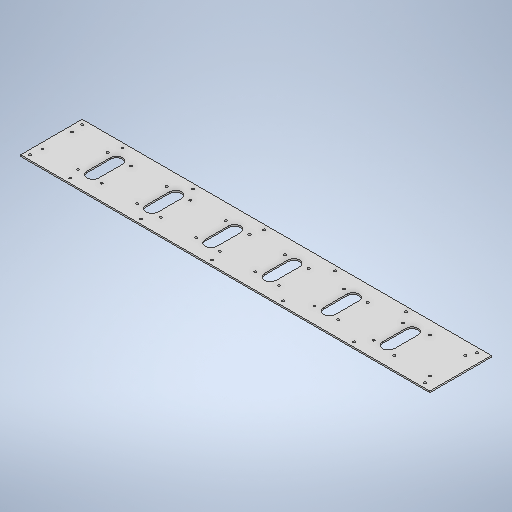
# Autodesk Inventor part: PCBMountingPlate
Saved by Autodesk Inventor 2025.1 (Build 291241000, 241)
## iProperties
Created: 2025-12-18
Part Number: PCBMountingPlate
Material: Generic
Document SubType Name: Modeling
Designer: Juxin
Density: 1 g/cm^3
Appearance: Default
Author: Juxin
Autodesk Inventor part; units mm, degrees
ref_plane "YZ Plane" through (0, 0, 0) normal (1, 0, 0) x (0, 1, 0)
ref_plane "XZ Plane" through (0, 0, 0) normal (0, 1, 0) x (-1, 0, 0)
ref_plane "XY Plane" through (0, 0, 0) normal (0, 0, 1) x (1, 0, 0)
sketch "Sketch1" plane through (0, 0, 0) normal (0, 1, 0) x (-1, 0, 0)
  line L0 (0, 0) -> (878.84, 0)
  line L1 (878.84, 0) -> (878.84, -66.04)
  line L2 (878.84, -66.04) -> (0, -66.04)
  line L3 (0, -66.04) -> (0, 0)
  line L4 (0, 0) -> (0, -20.32)
  line L5 (0, 0) -> (20.32, 0) construction
  line L6 (0, -20.32) -> (878.84, -20.32)
  line L7 (0, -10.16) -> (20.32, -10.16)
  line L8 (0, -10.16) -> (20.32, -10.16) construction
  circle A0 centre (20.32, -10.16) radius 2.54
  line L9 (20.32, -10.16) -> (172.72, -10.16)
  line L10 (20.32, -10.16) -> (172.72, -10.16) construction
  circle A1 centre (172.72, -10.16) radius 2.54
  line L11 (172.72, -10.16) -> (325.12, -10.16)
  circle A2 centre (325.12, -10.16) radius 2.54
  line L12 (325.12, -10.16) -> (477.52, -10.16)
  circle A3 centre (477.52, -10.16) radius 2.54
  line L13 (477.52, -10.16) -> (629.92, -10.16)
  circle A4 centre (629.92, -10.16) radius 2.54
  line L14 (629.92, -10.16) -> (782.32, -10.16)
  circle A5 centre (782.32, -10.16) radius 2.54
  line L15 (878.84, 0) -> (878.84, -10.16)
  line L16 (878.84, 0) -> (889, 0) construction
  line L17 (878.84, -10.16) -> (868.68, -10.16)
  circle A6 centre (868.68, -10.16) radius 2.54
  line L18 (0, 0) -> (0, -27.94)
  line L19 (0, 0) -> (27.94, 0) construction
  line L20 (0, -27.94) -> (27.94, -27.94)
  circle A7 centre (27.94, -27.94) radius 2.54
  line L21 (27.94, -27.94) -> (104.14, -27.94)
  line L22 (27.94, -27.94) -> (104.14, -27.94) construction
  circle A8 centre (104.14, -27.94) radius 2.54
  line L23 (104.14, -27.94) -> (129.54, -27.94)
  line L24 (142.24, -40.64) -> (142.24, -66.04)
  line L25 (142.24, -66.04) -> (116.84, -66.04)
  line L26 (116.84, -66.04) -> (116.84, -40.64)
  line L27 (116.84, -27.94) -> (116.84, -40.64)
  line L28 (116.84, -27.94) -> (129.54, -27.94) construction
  line L29 (116.84, -40.64) -> (129.54, -40.64)
  arc A9 (142.24, -40.64) -> (116.84, -40.64) centre (129.54, -40.64) ccw
  line L30 (142.24, -40.64) -> (154.94, -40.64) construction
  line L31 (142.24, -66.04) -> (154.94, -66.04)
  line L32 (142.24, -66.04) -> (154.94, -66.04) construction
  line L33 (154.94, -66.04) -> (154.94, -34.29)
  circle A10 centre (154.94, -34.29) radius 2.54
  line L34 (154.94, -34.29) -> (231.14, -34.29)
  line L35 (154.94, -34.29) -> (231.14, -34.29) construction
  circle A11 centre (231.14, -34.29) radius 2.54
  line L36 (154.94, -34.29) -> (104.14, -34.29)
  line L37 (154.94, -34.29) -> (205.74, -34.29) construction
  line L38 (269.24, -40.64) -> (269.24, -66.04)
  line L39 (243.84, -66.04) -> (243.84, -40.64)
  arc A12 (269.24, -40.64) -> (243.84, -40.64) centre (256.54, -40.64) ccw
  circle A13 centre (281.94, -34.29) radius 2.54
  line L40 (281.94, -34.29) -> (358.14, -34.29)
  circle A14 centre (358.14, -34.29) radius 2.54
  line L41 (281.94, -34.29) -> (231.14, -34.29)
  line L42 (396.24, -40.64) -> (396.24, -66.04)
  line L43 (370.84, -66.04) -> (370.84, -40.64)
  arc A15 (396.24, -40.64) -> (370.84, -40.64) centre (383.54, -40.64) ccw
  circle A16 centre (408.94, -34.29) radius 2.54
  line L44 (408.94, -34.29) -> (485.14, -34.29)
  circle A17 centre (485.14, -34.29) radius 2.54
  line L45 (408.94, -34.29) -> (358.14, -34.29)
  line L46 (523.24, -40.64) -> (523.24, -66.04)
  line L47 (497.84, -66.04) -> (497.84, -40.64)
  arc A18 (523.24, -40.64) -> (497.84, -40.64) centre (510.54, -40.64) ccw
  circle A19 centre (535.94, -34.29) radius 2.54
  line L48 (535.94, -34.29) -> (612.14, -34.29)
  circle A20 centre (612.14, -34.29) radius 2.54
  line L49 (535.94, -34.29) -> (485.14, -34.29)
  line L50 (650.24, -40.64) -> (650.24, -66.04)
  line L51 (624.84, -66.04) -> (624.84, -40.64)
  arc A21 (650.24, -40.64) -> (624.84, -40.64) centre (637.54, -40.64) ccw
  circle A22 centre (662.94, -34.29) radius 2.54
  line L52 (662.94, -34.29) -> (739.14, -34.29)
  circle A23 centre (739.14, -34.29) radius 2.54
  line L53 (662.94, -34.29) -> (612.14, -34.29)
  line L54 (777.24, -40.64) -> (777.24, -66.04)
  line L55 (751.84, -66.04) -> (751.84, -40.64)
  arc A24 (777.24, -40.64) -> (751.84, -40.64) centre (764.54, -40.64) ccw
  circle A25 centre (789.94, -34.29) radius 2.54
  line L56 (789.94, -34.29) -> (866.14, -34.29)
  circle A26 centre (866.14, -34.29) radius 2.54
  line L57 (789.94, -34.29) -> (739.14, -34.29)
  line L58 (0, -132.08) -> (878.84, -132.08)
  line L59 (878.84, -132.08) -> (878.84, -66.04)
  line L60 (0, -66.04) -> (0, -132.08)
  line L61 (0, -132.08) -> (0, -111.76)
  line L62 (0, -132.08) -> (20.32, -132.08) construction
  line L63 (0, -111.76) -> (878.84, -111.76)
  line L64 (0, -121.92) -> (20.32, -121.92)
  line L65 (0, -121.92) -> (20.32, -121.92) construction
  circle A27 centre (20.32, -121.92) radius 2.54
  line L66 (20.32, -121.92) -> (172.72, -121.92)
  line L67 (20.32, -121.92) -> (172.72, -121.92) construction
  circle A28 centre (172.72, -121.92) radius 2.54
  circle A29 centre (325.12, -121.92) radius 2.54
  line L68 (172.72, -121.92) -> (325.12, -121.92)
  circle A30 centre (477.52, -121.92) radius 2.54
  line L69 (325.12, -121.92) -> (477.52, -121.92)
  circle A31 centre (629.92, -121.92) radius 2.54
  line L70 (477.52, -121.92) -> (629.92, -121.92)
  circle A32 centre (782.32, -121.92) radius 2.54
  line L71 (629.92, -121.92) -> (782.32, -121.92)
  line L72 (878.84, -132.08) -> (878.84, -121.92)
  line L73 (878.84, -132.08) -> (889, -132.08) construction
  line L74 (878.84, -121.92) -> (868.68, -121.92)
  circle A33 centre (868.68, -121.92) radius 2.54
  line L75 (0, -132.08) -> (0, -104.14)
  line L76 (0, -132.08) -> (27.94, -132.08) construction
  line L77 (0, -104.14) -> (27.94, -104.14)
  circle A34 centre (27.94, -104.14) radius 2.54
  line L78 (27.94, -104.14) -> (104.14, -104.14)
  line L79 (27.94, -104.14) -> (104.14, -104.14) construction
  circle A35 centre (104.14, -104.14) radius 2.54
  line L80 (104.14, -104.14) -> (129.54, -104.14)
  line L81 (142.24, -91.44) -> (142.24, -66.04)
  line L82 (116.84, -66.04) -> (116.84, -91.44)
  line L83 (116.84, -104.14) -> (116.84, -91.44)
  line L84 (116.84, -104.14) -> (129.54, -104.14) construction
  line L85 (116.84, -91.44) -> (129.54, -91.44)
  arc A36 (116.84, -91.44) -> (142.24, -91.44) centre (129.54, -91.44) ccw
  line L86 (142.24, -91.44) -> (154.94, -91.44) construction
  line L87 (154.94, -66.04) -> (154.94, -97.79)
  circle A37 centre (154.94, -97.79) radius 2.54
  line L88 (154.94, -97.79) -> (231.14, -97.79)
  line L89 (154.94, -97.79) -> (231.14, -97.79) construction
  circle A38 centre (231.14, -97.79) radius 2.54
  line L90 (154.94, -97.79) -> (104.14, -97.79)
  line L91 (154.94, -97.79) -> (205.74, -97.79) construction
  line L92 (281.94, -97.79) -> (231.14, -97.79)
  line L93 (281.94, -97.79) -> (358.14, -97.79)
  line L94 (269.24, -91.44) -> (269.24, -66.04)
  line L95 (243.84, -66.04) -> (243.84, -91.44)
  arc A39 (243.84, -91.44) -> (269.24, -91.44) centre (256.54, -91.44) ccw
  circle A40 centre (281.94, -97.79) radius 2.54
  circle A41 centre (358.14, -97.79) radius 2.54
  line L96 (408.94, -97.79) -> (358.14, -97.79)
  line L97 (408.94, -97.79) -> (485.14, -97.79)
  line L98 (396.24, -91.44) -> (396.24, -66.04)
  line L99 (370.84, -66.04) -> (370.84, -91.44)
  arc A42 (370.84, -91.44) -> (396.24, -91.44) centre (383.54, -91.44) ccw
  circle A43 centre (408.94, -97.79) radius 2.54
  circle A44 centre (485.14, -97.79) radius 2.54
  line L100 (535.94, -97.79) -> (485.14, -97.79)
  line L101 (535.94, -97.79) -> (612.14, -97.79)
  line L102 (523.24, -91.44) -> (523.24, -66.04)
  line L103 (497.84, -66.04) -> (497.84, -91.44)
  arc A45 (497.84, -91.44) -> (523.24, -91.44) centre (510.54, -91.44) ccw
  circle A46 centre (535.94, -97.79) radius 2.54
  circle A47 centre (612.14, -97.79) radius 2.54
  line L104 (662.94, -97.79) -> (612.14, -97.79)
  line L105 (662.94, -97.79) -> (739.14, -97.79)
  line L106 (650.24, -91.44) -> (650.24, -66.04)
  line L107 (624.84, -66.04) -> (624.84, -91.44)
  arc A48 (624.84, -91.44) -> (650.24, -91.44) centre (637.54, -91.44) ccw
  circle A49 centre (662.94, -97.79) radius 2.54
  circle A50 centre (739.14, -97.79) radius 2.54
  line L108 (789.94, -97.79) -> (739.14, -97.79)
  line L109 (789.94, -97.79) -> (866.14, -97.79)
  line L110 (777.24, -91.44) -> (777.24, -66.04)
  line L111 (751.84, -66.04) -> (751.84, -91.44)
  arc A51 (751.84, -91.44) -> (777.24, -91.44) centre (764.54, -91.44) ccw
  circle A52 centre (789.94, -97.79) radius 2.54
  circle A53 centre (866.14, -97.79) radius 2.54
  dimension "d8" = 878.84
  dimension "d9" = 66.04
  dimension "d10" = 20.32
  dimension "d11" = 90
  dimension "d12" = 878.84
  dimension "d14" = 20.32
  dimension "d15" = 0
  dimension "d16" = 5.08
  dimension "d17" = 152.4
  dimension "d19" = 5.08
  dimension "d20" = 152.4
  dimension "d21" = 5.08
  dimension "d22" = 152.4
  dimension "d23" = 5.08
  dimension "d24" = 152.4
  dimension "d25" = 5.08
  dimension "d26" = 152.4
  dimension "d27" = 5.08
  dimension "d28" = 10.16
  dimension "d29" = 90
  dimension "d30" = 10.16
  dimension "d31" = 90
  dimension "d32" = 5.08
  dimension "d33" = 27.94
  dimension "d34" = 90
  dimension "d35" = 27.94
  dimension "d36" = 90
  dimension "d37" = 5.08
  dimension "d38" = 76.2
  dimension "d39" = 0
  dimension "d40" = 5.08
  dimension "d41" = 25.4
  dimension "d43" = 25.4
  dimension "d46" = 12.7
  dimension "d47" = 90
  dimension "d48" = 12.7
  dimension "d51" = 12.7
  dimension "d52" = 0
  dimension "d53" = 31.75
  dimension "d54" = 90
  dimension "d55" = 5.08
  dimension "d56" = 76.2
  dimension "d57" = 0
  dimension "d58" = 5.08
  dimension "d59" = 50.8
  dimension "d60" = 180
  dimension "d61" = 25.4
  dimension "d62" = 5.08
  dimension "d63" = 76.2
  dimension "d64" = 5.08
  dimension "d65" = 50.8
  dimension "d66" = 25.4
  dimension "d67" = 5.08
  dimension "d68" = 76.2
  dimension "d69" = 5.08
  dimension "d70" = 50.8
  dimension "d71" = 25.4
  dimension "d72" = 5.08
  dimension "d73" = 76.2
  dimension "d74" = 5.08
  dimension "d75" = 50.8
  dimension "d76" = 25.4
  dimension "d77" = 5.08
  dimension "d78" = 76.2
  constraints: 224 end point, 85 symmetric about line, 54 centre point, 26 horizontal, 26 point on circle, 16 coincident, 10 equal length, 8 parallel, 7 perpendicular, 4 collinear, 2 midpoint, 1 vertical, 27 other
  measures "d8" distance of L1.end L2.end
  measures "d9" distance of L0.end L1.end
  measures "d10" distance of L0.start L4.end
  measures "d11" angle of L4 L5
  measures "d12" distance of L4.end L6.end
  measures "d14" distance of L7.start L7.end
  measures "d15" distance between parallel lines of L7 L8
  measures "d16" diameter of A0
  measures "d17" distance of L9.start L9.end
  measures "d19" diameter of A1
  measures "d20" distance of L11.start L11.end
  measures "d21" diameter of A2
  measures "d22" distance of L12.start L12.end
  measures "d23" diameter of A3
  measures "d24" distance of L13.start L13.end
  measures "d25" diameter of A4
  measures "d26" distance of L14.start L14.end
  measures "d27" diameter of A5
  measures "d28" distance of L0.end L15.end
  measures "d29" angle of L15 L16
  measures "d30" distance of L15.end L17.end
  measures "d31" angle of L15 L17
  measures "d32" diameter of A6
  measures "d33" distance of L0.start L18.end
  measures "d34" angle of L18 L19
  measures "d35" distance of L18.end L20.end
  measures "d36" angle of L20 L18
  measures "d37" diameter of A7
  measures "d38" distance of L21.start L21.end
  measures "d39" distance between parallel lines of L21 L22
  measures "d40" diameter of A8
  measures "d41" distance of L23.start L23.end
  measures "d43" distance of L24.start L24.end
  measures "d46" distance of L26.end L29.end
  measures "d47" angle of L29 L27
  measures "d48" distance of L27.start L26.end
  measures "d51" distance of L24.end L31.end
  measures "d52" distance between parallel lines of L31 L32
  measures "d53" distance of L31.end L33.end
  measures "d54" angle of L33 L31
  measures "d55" diameter of A10
  measures "d56" distance of L34.start L34.end
  measures "d57" distance between parallel lines of L34 L35
  measures "d58" diameter of A11
  measures "d59" distance of L34.start L36.end
  measures "d60" angle of L36 L37
  measures "d61" distance of L38.start L38.end
  measures "d62" diameter of A13
  measures "d63" distance of L41.start L40.end
  measures "d64" diameter of A14
  measures "d65" distance of L41.start L41.end
  measures "d66" distance of L42.start L42.end
  measures "d67" diameter of A16
  measures "d68" distance of L45.start L44.end
  measures "d69" diameter of A17
  measures "d70" distance of L45.start L45.end
  measures "d71" distance of L46.start L46.end
  measures "d72" diameter of A19
  measures "d73" distance of L49.start L48.end
  measures "d74" diameter of A20
  measures "d75" distance of L49.start L49.end
  measures "d76" distance of L50.start L50.end
  measures "d77" diameter of A22
  measures "d78" distance of L53.start L52.end
extrude "Extrusion1" add sketch "Sketch1" along normal blind 3.175 contours L0 L1 L6 L3 | L6 L1 L2 L54 A24 L57 A23 L52 A22 L53 A21 A20 L48 A19 L49 A18 A17 L44 A16 L45 A15 A14 L40 A13 L41 A12 A11 L34 A10 L36 A9 L23 A8 L21 A7 L20 L3 | L20 A7 L21 A8 L23 L27 L26 L2 L3 | L59 L63 L60 L77 A34 L78 A35 L80 A36 L90 A37 L88 A38 L92 A39 A40 L93 A41 L96 A42 A43 L97 A44 L100 A45 A46 L101 A47 L104 A48 A49 L105 A50 L108 A51 L110 L2 | L2 L82 L83 L80 A35 L78 A34 L77 L60 | L59 L58 L60 L63 | L111 A51 L108 A50 L105 A49 L104 A48 L106 L2 | L2 L50 A21 L53 A22 L52 A23 L57 A24 L55 | L24 A9 L36 A10 L33 L2 | L2 L87 A37 L90 A36 L81 | L27 L36 A9 | A36 L90 L83 | L33 A10 L34 A11 L41 A12 L39 L2 | L2 L95 A39 L92 A38 L88 A37 L87 | L27 L23 A9 L36 | L90 A36 L80 L83 | L107 A48 L104 A47 L101 A46 L100 A45 L102 L2 | L2 L46 A18 L49 A19 L48 A20 L53 A21 L51 | L38 A12 L41 A13 L40 A14 L45 A15 L43 L2 | L2 L99 A42 L96 A41 L93 A40 L92 A39 L94 | L103 A45 L100 A44 L97 A43 L96 A42 L98 L2 | L2 L42 A15 L45 A16 L44 A17 L49 A18 L47
body "Solid1"
